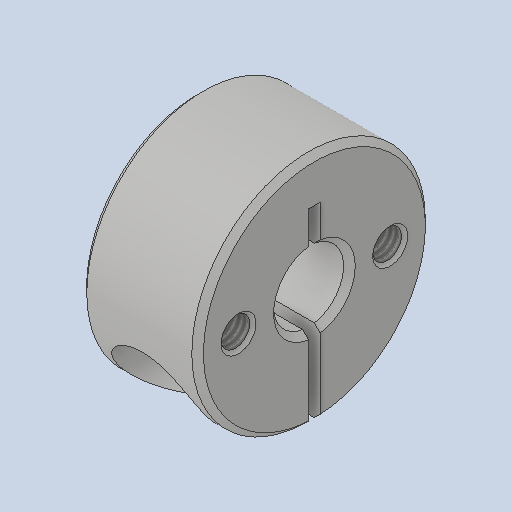
# Autodesk Inventor part: SCSW6-10b
Saved by Autodesk Inventor 2025.2 (Build 292293000, 293)
## iProperties
Created: 2024-08-14
Part Number: SCSW6-10b
Material: Generic
Catalog Web Link: www.cadenas.de
Description: SCSW, PSCSW, SSCSW, SCSWA, SCSWAW-b-Set Collars - Slit 2 Hole/2 Tap - Standard Type - 2 Tap Type
Vendor: MISUMI
Document SubType Name: Modeling
Designer: psAdmin
Manufacturer: MISUMI
Mass: 2.36227 g
Surface Area: 17.7233 cm^2
Volume: 2.36227 cm^3
Density: 1 g/cm^3
Appearance: PSOLRGB-175-175-175
Category: PARTsolutions
Company: MISUMI
PSOL_IDENT_0: {$CADENAS_DATA/23d-libs/misumi/metric/03_set_collars/scsw_b.prj},199 {VTYP=3D},{NB=SCSW6-10b},{LINA=
PSOL_IDENT_1: SCSW6-10b},{NN=SCSW, PSCSW, SSCSW, SCSWA, SCSWAW-b},{DATE=30.11.2021 05:42:06},{GEOMDATE=15.09.2021
PSOL_IDENT_2: 06:01:21},{VERSION=},{LINEID=220},{WBVAR=MAT,ST,BS},{WBNUMERIC=BS}  {NB=SCSW6-10b},{LINA=SCSW6-10b},
PSOL_IDENT_3: {KT=DUMMY},{PN=SCSW6-10},{TYPE=SCSW},{MAT=1045},{MATA='1045','S45C Equivalent','304','SUS304 Equival
PSOL_IDENT_4: ent','2017','2017 Aluminum Alloy'},{ST=Black Oxide},{AC=Hexagon Socket Head Set Screw 1 Pc.},{D=6},{
PSOL_IDENT_5: BS=10},{B1=8,10},{D1=20},{M=M4},{THMD=4},{THDMIN=3.242},{ST0='Black Oxide','Black Oxide','Electroles
PSOL_IDENT_6: s Nickel Plating','Electroless Nickel Plating'},{DD=4.5},{R=3.75},{W=1.0},{X=6.0},{Y=4.0},{Z=6~6.5},
PSOL_IDENT_7: {S=3.5},{P=13},{C=0.5},{L=10},{M1=M3},{ZZ=6.25},{THMD1=3},{THDMIN1=2.459}
NB: SCSW6-10b
NN: SCSW, PSCSW, SSCSW, SCSWA, SCSWAW-b
NT: Set Collars - Slit 2 Hole/2 Tap - Standard Type - 2 Tap Type
NBSYN: $PN.b
LINA: SCSW6-10b
CATALOG: Misumi
PN: SCSW6-10
MAT: S45C Equivalent
ST: Black Oxide
AC: Hexagon Socket Head Set Screw 1 Pc.
D: 6
BS: 10
D1: 20
M: M4
DD: 4.5
R: 3.75
W: 1
X: 6
Y: 4
Z: 6~6.5
S: 3.5
P: 13
M1: M3
SUPPLIER: MISUMI
ARTICLENO: SCSW6-10b
BOMINFO: SCSW6-10b
CREATOR: CADENAS GmbH
Title: SCSW6-10b
Author: Cadenas PARTsolutions
Comments: Set Collars - Slit 2 Hole/2 Tap - Standard Type - 2 Tap Type
Autodesk Inventor part; units mm, degrees
sketch "Sketch_1" plane through (0, 0, 0) normal (0, 0, 1) x (1, 0, 0)
  line L0 (5, 0) -> (-5, 0)
  line L1 (-5, 9.5) -> (-5, 3.5)
  line L2 (-5, 3.5) -> (-4.5, 3)
  line L3 (-4.5, 3) -> (4.5, 3)
  line L4 (4.5, 3) -> (5, 3.5)
  line L5 (5, 3.5) -> (5, 9.5)
  line L6 (5, 9.5) -> (4.5, 10)
  line L7 (4.5, 10) -> (-4.5, 10)
  line L8 (-4.5, 10) -> (-5, 9.5)
  constraints: 18 end point
revolve "Revolution1" add sketch "Sketch_1" angle 360 about axis through (5, 0, 0) along (1, 0, 0)
sketch "Sketch_2" plane through (0, 0, 0) normal (1, 0, 0) x (0, 1, 0)
  line L0 (-10, 0.5) -> (-10, -0.5)
  line L1 (-10, -0.5) -> (6.25, -0.5)
  line L2 (6.25, -0.5) -> (6.25, 0.5)
  line L3 (6.25, 0.5) -> (-10, 0.5)
  constraints: 8 end point
extrude "Extrusion1" cut sketch "Sketch_2" along normal mid plane 10
sketch "Sketch_3" plane through (0, 0, 0) normal (1, 0, 0) x (0, 1, 0)
  line L0 (-6, 10) -> (-6, 0)
  line L1 (-6, 0) -> (-8.25, 0)
  line L2 (-8.25, 0) -> (-8.25, 4)
  line L3 (-8.25, 4) -> (-9.75, 4)
  line L4 (-9.75, 4) -> (-9.75, 10)
  line L5 (-9.75, 10) -> (-6, 10)
  line L6 (-6, 10) -> (-6, 0)
  constraints: 14 end point
revolve "Revolution2" cut sketch "Sketch_3" angle 360 about axis through (0, -6, 10) along (0, 0, 1)
sketch "Sketch_4" plane through (0, 0, 0) normal (1, 0, 0) x (0, 1, 0)
  line L0 (-6, -9.5) -> (-6, -0.5)
  line L1 (-6, -0.5) -> (-4, -0.5)
  line L2 (-4, -0.5) -> (-4.379, -0.879)
  line L3 (-4.379, -0.879) -> (-4.379, -9.5)
  line L4 (-4.379, -9.5) -> (-6, -9.5)
  line L5 (-6, -9.5) -> (-6, -0.5)
  constraints: 12 end point
revolve "Revolution3" cut sketch "Sketch_4" angle 360 about axis through (0, -6, -9.5) along (0, 0, -1)
thread "Thread1" size "M4x0.7" class "6H" standard "ISO Metric profile" length 8.2861
sketch "Sketch_7" plane through (0, 0, -6.5) normal (0, 0, 1) x (1, 0, 0)
  line L0 (5, 0) -> (-5, 0)
  line L1 (-5, 0) -> (-5, 1.5)
  line L2 (-5, 1.5) -> (-4.7295, 1.2295)
  line L3 (-4.7295, 1.2295) -> (4.7295, 1.2295)
  line L4 (4.7295, 1.2295) -> (5, 1.5)
  line L5 (5, 1.5) -> (5, 0)
  line L6 (5, 0) -> (-5, 0)
  constraints: 14 end point
revolve "Revolution4" cut sketch "Sketch_7" angle 360 about axis through (5, 0, -6.5) along (1, 0, 0)
thread "Thread2" size "M3x0.5" class "6H" standard "ISO Metric profile" full length
sketch "Sketch_8" plane through (0, 0, 6.5) normal (0, 0, 1) x (1, 0, 0)
  line L0 (5, 0) -> (-5, 0)
  line L1 (-5, 0) -> (-5, 1.5)
  line L2 (-5, 1.5) -> (-4.7295, 1.2295)
  line L3 (-4.7295, 1.2295) -> (4.7295, 1.2295)
  line L4 (4.7295, 1.2295) -> (5, 1.5)
  line L5 (5, 1.5) -> (5, 0)
  line L6 (5, 0) -> (-5, 0)
  constraints: 14 end point
revolve "Revolution5" cut sketch "Sketch_8" angle 360 about axis through (5, 0, 6.5) along (1, 0, 0)
thread "Thread3" size "M3x0.5" class "6H" standard "ISO Metric profile" full length
ref_plane "body_screw_XY" through (0, -6, 4) normal (0, 0, 1) x (1, 0, 0)
ref_plane "body_screw_YZ" through (0, -6, 4) normal (1, 0, 0) x (0, 1, 0)
ref_plane "body_screw_ZX" through (0, -6, 4) normal (0, 1, 0) x (0, 0, 1)
body "Solid1"
